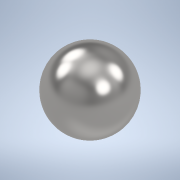
# Autodesk Inventor part: BearingBall
Saved by Autodesk Inventor 2020 (Build 240168000, 168)
## iProperties
Created: 2020-01-04
Part Number: BearingBall
Material: Steel, Carbon
Document SubType Name: Modeling
Designer: Connor
Density: 7.85 g/cm^3
Appearance: Semi-Polished
Author: Connor
Autodesk Inventor part; units mm, degrees
ref_plane "YZ Plane" through (0, 0, 0) normal (1, 0, 0) x (0, 1, 0)
ref_plane "XZ Plane" through (0, 0, 0) normal (0, 1, 0) x (-1, 0, 0)
ref_plane "XY Plane" through (0, 0, 0) normal (0, 0, 1) x (1, 0, 0)
sketch "Sketch1" plane through (0, 0, 0) normal (0, 0, 1) x (1, 0, 0)
  arc A0 (0, -1.5875) -> (0, 1.5875) centre (0, 0) ccw
  line L0 (0, 1.5875) -> (0, -1.5875)
  dimension "d0" = 1.5875
  constraints: 2 end point, 2 point on circle, 1 centre point, 1 coincident, 1 midpoint, 1 vertical
  measures "d0" radius of A0
revolve "Revolution1" add sketch "Sketch1" angle 360 about axis through (0, 1.5875, 0) along (0, -1, 0)
body "Solid1"
